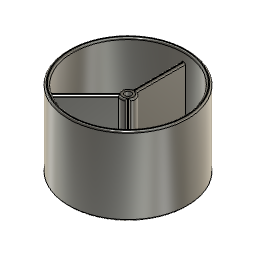
Part_wheel v1 (Autodesk Fusion 360 design; units mm, degrees)
Autodesk Fusion 360 part; units mm, degrees
sketch "Sketch1" plane through (0, 0, 0) normal (0, 0, 1) x (1, 0, 0)
  circle A0 centre (0, 0) radius 76.2
  circle A1 centre (0, 0) radius 71.2
  circle A2 centre (0, 0) radius 9
  circle A3 centre (0, 0) radius 4.1
  line L0 (0, 0) -> (0, 76.2) construction
  line L1 (0, 0) -> (53.8815, -53.8815) construction
  line L2 (0, 0) -> (76.2, 0) construction
  line L3 (0, 0) -> (-53.745, -53.745) construction
  line L4 (0, 0) -> (76.007, 0) construction
  line L5 (2.5, 76.159) -> (2.5, 1.7375)
  line L6 (-2.5, 76.159) -> (-2.5, 0.6433)
  line L7 (55.6203, -52.0848) -> (2.1883, 1.3473)
  line L8 (55.6203, -52.0848) -> (131.2596, -52.0848) construction
  line L9 (52.0848, -55.6203) -> (-0.8288, -2.7067)
  line L10 (-55.6203, -52.0848) -> (-2.626, 0.9096)
  line L11 (-55.6203, -52.0848) -> (18.9248, -52.0848) construction
  line L12 (-52.0848, -55.6203) -> (1.7678, -1.7678)
  dimension "d1" = 152.4
  dimension "d2" = 142.4
  dimension "d3" = 18
  dimension "d4" = 8.2
  dimension "d5" = 45
  dimension "d6" = 135
  dimension "d7" = 135
  dimension "d8" = 75.5643
  dimension "d9" = 45
  dimension "d10" = 2.5
  dimension "d11" = 2.5
  dimension "d12" = 2.5
  dimension "d13" = 2.5
  dimension "d14" = 2.5
  dimension "d15" = 2.5
  constraint coincident A0.centre A1.centre
  constraint concentric A0 A1
  constraint concentric A0 A2
  constraint concentric A0 A3
  constraint coincident A0 L0.end
  constraint vertical L0
  constraint horizontal L2
  constraint horizontal L4
  constraint coincident A0 L5.start
  constraint perpendicular L2 L5
  constraint coincident A0 L6.start
  constraint parallel L0 L6
  constraint horizontal L8
  constraint coincident A0 L7.start
  constraint coincident A0 L9.start
  constraint parallel L1 L9
  constraint horizontal L11
  constraint coincident A0 L10.start
  constraint coincident A0 L12.start
  constraint coincident L1 L12.end
  constraint perpendicular L1 L12
  measures "d1" diameter of A0
  measures "d2" diameter of A1
  measures "d3" diameter of A2
  measures "d4" diameter of A3
  measures "d5" angle of L1 L2
  measures "d6" angle of L3 L4
  measures "d7" angle of L7 L8
  measures "d8" distance of L7.start L7.end
  measures "d9" angle of L10 L11
  measures "d10" distance of L0 L5
  measures "d11" distance of L0 L6
  measures "d12" distance of L3 L10
  measures "d13" distance of L3 L12
  measures "d14" distance of L1 L7
  measures "d15" distance of L1 L9
extrude "Extrude1" add sketch "Sketch1" along normal blind 50 and the other way blind 50 contours A0 A1 L5 L7 | A0 A1 L5 L6 | A0 A1 L7 L9 | A0 A1 L6 L10 | A0 A1 L9 L12 | A0 A1 L10 L12
extrude "Extrude2" add sketch "Sketch1" along normal blind 38 and the other way blind 38 contours A1 A2 L5 L6 | A1 A2 L7 L9 | A2 A3 L5 L6 | A2 A3 L5 L7 | A2 A3 L7 L9 | A1 A2 L10 L12 | A2 A3 L6 L10 | A2 A3 L9 L12 | A2 A3 L10 L12
fillet "Fillet1" radius 2 2 edges at (-71.0433, -27.5551, 50) (-66.3817, 25.747, 50)
fillet "Fillet2" radius 2 2 edges at (-71.0433, 27.5551, -50) (-66.3817, -25.747, -50)
fillet "Fillet3" radius 2 9 edges at (2.5, 39.901, 38) (-2.5, 39.901, 38) (-29.982, -26.4465, 38) (-26.4465, -29.982, 38) (26.4465, -29.982, 38) (29.982, -26.4465, 38) (8.3149, 3.4442, 38) (0, -9, 38) (-8.3149, 3.4442, 38)
fillet "Fillet4" radius 2 9 edges at (29.982, -26.4465, -38) (26.4465, -29.982, -38) (8.3149, 3.4442, -38) (0, -9, -38) (-26.4465, -29.982, -38) (-29.982, -26.4465, -38) (-8.3149, 3.4442, -38) (-2.5, 39.901, -38) (2.5, 39.901, -38)
